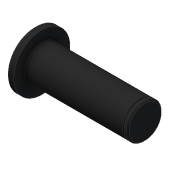
# Autodesk Inventor part: Boltx50
Saved by Autodesk Inventor 2020.1 (Build 241239000, 239)
## iProperties
Part Number: Boltx50
Document SubType Name: Modeling
Created: 2003-03-06
Material: Standard
Designer: rueghs
Density: 1 g/cm^3
Appearance: Brokk_Gray
Control State: 0
Master: False
Checked Out: False
Shininess: 64.0
Length Units: 11269
Angle Units: 11279
Time Units: 11290
Mass Units: 11283
Length Display Precision: 3
Angle Display Precision: 2
Compacted: True
Density: 0.0
Volumn: 0.0
Area: 0.0
PropertySet Name: Model Information
Author: rueghs
Autodesk Inventor part; units mm, degrees
ref_plane "YZ Plane" through (0, 0, 0) normal (1, 0, 0) x (0, 1, 0)
ref_plane "XZ Plane" through (0, 0, 0) normal (0, 1, 0) x (-1, 0, 0)
ref_plane "XY Plane" through (0, 0, 0) normal (0, 0, 1) x (1, 0, 0)
sketch "Skizze1" plane through (0, 0, 0) normal (0, 0, 1) x (1, 0, 0)
  line L0 (-70, 25) -> (-70, 40)
  line L1 (-70, 40) -> (-80, 40)
  line L2 (-80, 40) -> (-80, 0)
  line L3 (-80, 0) -> (77, 0)
  line L4 (77, 0) -> (77, 25)
  line L5 (72, 25) -> (72, 23)
  line L6 (72, 23) -> (70, 23)
  line L7 (70, 23) -> (70, 25)
  line L8 (77, 25) -> (72, 25)
  line L9 (70, 25) -> (-70, 25)
  dimension "d0" = 80
  dimension "d1" = 10
  dimension "d2" = 50
  dimension "d3" = 46
  dimension "d7" = 2
  dimension "d8" = 5
  dimension "d13" = 140
  constraints: 20 end point, 4 parallel, 3 perpendicular, 2 horizontal, 1 collinear
  measures "d0" diameter of L1 L3
  measures "d1" distance of L0.end L1.end
  measures "d2" diameter of L9 L3
  measures "d3" diameter of L6 L3
  measures "d7" distance of L5.end L6.end
  measures "d8" distance of L4.end L5.start
  measures "d13" distance of L7.end L0.start
revolve "Drehung1" add sketch "Skizze1" angle 360 about axis through (-80, 0, 0) along (1, 0, 0)
chamfer "Fase1" distance 2 angle 45 1 edges at (-80, -40, 0)
chamfer "Fase2" distance 2 angle 45 1 edges at (77, -25, 0)
body "Solid1"
